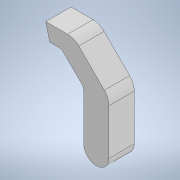
# Autodesk Inventor part: switch-pusher
Saved by Autodesk Inventor 2021 (Build 250183000, 183)
## iProperties
Created: 2024-05-24
Part Number: switch-pusher
Material: Generic
Document SubType Name: Modeling
Designer: Toby
Density: 1 g/cm^3
Appearance: Default
Author: Toby
Autodesk Inventor part; units mm, degrees
ref_plane "YZ Plane" through (0, 0, 0) normal (1, 0, 0) x (0, 1, 0)
ref_plane "XZ Plane" through (0, 0, 0) normal (0, 1, 0) x (-1, 0, 0)
ref_plane "XY Plane" through (0, 0, 0) normal (0, 0, 1) x (1, 0, 0)
sketch "Sketch2" plane through (0, 0, 0) normal (0, 0, 1) x (1, 0, 0)
  circle A0 centre (0, 0) radius 4
  line L0 (-4, 0) -> (4, 0)
  line L1 (4, 0) -> (4, 25)
  line L2 (4, 25) -> (-4, 25)
  line L3 (-4, 25) -> (-4, 0)
  point P0 (4, 0)
  dimension "d11" = 8
  dimension "d12" = 8
  dimension "d13" = 25
  constraints: 8 end point, 2 parallel, 1 coincident, 1 horizontal, 1 perpendicular, 3 other
  measures "d12" distance of L2.end L1.end
  measures "d13" distance of L1.end L0.end
extrude "Extrusion2" add sketch "Sketch2" along normal blind 5
sketch "Sketch3" plane through (0, 0, 5) normal (0, 0, 1) x (1, 0, 0)
  line L0 (4, 0) -> (4, 25) projected
  line L1 (-16, 27.5) -> (4, 27.5)
  line L2 (4, 27.5) -> (4, 22.5)
  line L3 (4, 22.5) -> (-16, 22.5)
  line L4 (-16, 22.5) -> (-16, 27.5)
  line L5 (4, 25) -> (-4, 25) projected
  point P0 (0, 0)
  point P1 (3, 25)
  dimension "d16" = 2.5
  dimension "d17" = 2.5
  dimension "d18" = 20
  constraints: 8 end point, 2 parallel, 1 horizontal, 1 perpendicular, 1 point on line
  measures "d16" distance between parallel lines of L5 L1
  measures "d17" distance between parallel lines of L5 L3
  measures "d18" distance between parallel lines of L2 L4
extrude "Extrusion3" add sketch "Sketch3" against normal blind 5
sketch "Sketch4" plane through (0, 0, 5) normal (0, 0, 1) x (1, 0, 0)
  line L0 (4, 0) -> (4, 27.5) projected
  line L1 (-16, 22.5) -> (-16, 27.5) projected
  line L2 (4, 27.5) -> (-16, 27.5)
  line L3 (-16, 27.5) -> (-16, 22.5)
  line L4 (-16, 22.5) -> (4, 22.5)
  line L5 (4, 22.5) -> (4, 27.5)
  point P0 (0, 0)
  constraints: 8 end point, 2 parallel, 1 horizontal, 1 perpendicular
extrude "Extrusion4" add sketch "Sketch4" along normal blind 3
sketch "Sketch6" plane through (0, 0, 0) normal (0, 0, -1) x (-1, 0, 0)
  circle A0 centre (0, 0) radius 3.5
  dimension "d30" = 7
  constraints: 1 centre point, 1 coincident
  measures "d30" diameter of A0
extrude "Extrusion6" cut sketch "Sketch6" against normal blind 5
sketch "Sketch7" plane through (0, 0, 0) normal (0, 0, -1) x (-1, 0, 0)
  line L0 (-3.2, -6) -> (3.2, -6)
  line L1 (3.2, -6) -> (3.2, -1)
  line L2 (3.2, -1) -> (-3.2, -1)
  line L3 (-3.2, -1) -> (-3.2, -6)
  line L4 (-4, 0) -> (-4, 27.5) projected
  line L5 (4, 22.5) -> (4, 0) projected
  point P0 (0, 0)
  point P1 (-4, 24.5)
  dimension "d33" = 1
  dimension "d34" = 6
  dimension "d35" = 0.8
  dimension "d36" = 0.8
  constraints: 8 end point, 2 parallel, 1 horizontal, 1 perpendicular
  measures "d33" distance from line of point (0, 0) L2
  measures "d34" distance from line of L0 point (0, 0)
  measures "d35" distance between parallel lines of L3 L4
  measures "d36" distance between parallel lines of L1 L5
extrude "Extrusion7" cut sketch "Sketch7" against normal blind 5
sketch "Sketch8" plane through (0, 0, 0) normal (0, 0, -1) x (-1, 0, 0)
  circle A0 centre (0, 16) radius 2.1
  arc A1 (3.2, -1.4177) -> (-3.2, -1.4177) centre (0, 0) ccw projected
  line L0 (-3.5, 0) -> (-2.1, 16)
  line L1 (2.1, 16) -> (3.4864, 0.308)
  point P0 (-3.4468, 0.6078)
  dimension "d39" = 16
  dimension "d40" = 4.2
  constraints: 4 end point, 4 point on circle, 1 centre point, 1 coincident, 1 tangent
  measures "d39" distance of point (0, 0) point (0, 16)
  measures "d40" diameter of A0
extrude "Extrusion8" cut sketch "Sketch8" against normal blind 5 contours A0 | L1 A1 L0 A0
sketch "Sketch10" plane through (0, 0, 5) normal (0, 0, 1) x (1, 0, 0)
  line L0 (-4, 22.5) -> (-4, 0) projected
  line L1 (4, 0) -> (4, 22.5) projected
  line L2 (-4, 22.5) -> (4, 22.5)
  line L3 (4, 22.5) -> (4, 0)
  line L4 (4, 0) -> (-4, 0)
  line L5 (-4, 0) -> (-4, 22.5)
  point P0 (0, 0)
  point P1 (-4, 15.5)
  point P2 (-4, 15.5)
  point P3 (-4, 14.5)
  constraints: 8 end point, 2 parallel, 1 horizontal, 1 perpendicular
extrude "Extrusion10" add sketch "Sketch10" along normal blind 3
chamfer "Chamfer5" distance 7 angle 45 1 edges at (-4, 22.5, 4)
chamfer "Chamfer6" distance 11 angle 45 1 edges at (4, 27.5, 4)
fillet "Fillet6" radius 5 2 edges at (-7, 27.5, 4) (4, 16.5, 4)
fillet "Fillet7" radius 2 2 edges at (-11, 22.5, 4) (-4, 15.5, 4)
sketch "Sketch14" plane through (0, 0, 5) normal (0, 0, 1) x (1, 0, 0)
  circle A0 centre (0, 0) radius 4
  constraints: 1 centre point, 1 coincident
extrude "Extrusion14" add sketch "Sketch14" along normal blind 3
sketch "Sketch15" plane through (0, 0, 8) normal (0, 0, 1) x (1, 0, 0)
  line L0 (-16, 22.5) -> (-16, 27.5) projected
  line L1 (-16, 27.5) -> (-16, 22.5)
  line L2 (-16, 22.5) -> (-14.7, 22.5)
  line L3 (-11.8284, 22.5) -> (-16, 22.5) projected
  line L4 (-16, 27.5) -> (-14.7, 22.5)
  point P0 (0, 0)
  dimension "d82" = 1.3
  constraints: 6 end point, 1 collinear, 1 point on line
  measures "d82" distance of L0.start L2.end
extrude "Extrusion15" cut sketch "Sketch15" against normal blind 20
body "Solid2"
